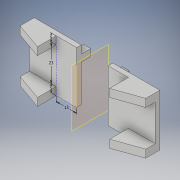
# Autodesk Inventor part: turret_servo_grip
Saved by Autodesk Inventor 2019 (Build 230136000, 136)
## iProperties
Created: 2019-04-21
Part Number: turret_servo_grip
Material: Ogólny
Document SubType Name: Modeling
Designer: terg
Density: 1 g/cm^3
Appearance: Domyślna
Author: terg
Autodesk Inventor part; units mm, degrees
ref_plane "XZ Plane" through (0, 0, 0) normal (0, 1, 0) x (-1, 0, 0)
ref_plane "XY Plane" through (0, 0, 0) normal (0, 0, 1) x (1, 0, 0)
sketch "Szkic1" plane through (0, 0, 0) normal (0, 0, 1) x (1, 0, 0)
  point P0 (0, 0)
sketch "Szkic2" plane through (0, 0, 0) normal (0, 0, 1) x (1, 0, 0)
  line L0 (0, 0) -> (-4.5, 0)
  line L1 (-4.5, 0) -> (-4.5, 4.5)
  line L2 (-4.5, 4.5) -> (0, 4.5)
  line L3 (0, 4.5) -> (0, 0)
  dimension "d0" = 4.5
  dimension "d1" = 4.5
  constraints: 8 end point, 2 parallel, 1 horizontal, 1 perpendicular
  measures "d0" distance of L1.end L2.end
  measures "d1" distance of L0.end L1.end
extrude "Wyciągnięcie proste1" add sketch "Szkic2" along normal blind 6
sketch "Szkic3" plane through (0, 0, 6) normal (0, 0, 1) x (1, 0, 0)
  line L0 (0, 0) -> (0, 4.5) projected
  line L1 (0, 4.5) -> (0, 9.5)
  line L2 (0, 9.5) -> (-30, 9.5)
  line L3 (-30, 9.5) -> (-30, -23.5)
  line L4 (-30, -23.5) -> (0, -23.5)
  line L5 (0, -23.5) -> (0, 9.5)
  point P0 (-4.5, 0)
  dimension "d7" = 5
  dimension "d8" = 30
  dimension "d9" = 33
  constraints: 10 end point, 2 parallel, 1 horizontal, 1 perpendicular, 1 vertical
  measures "d7" distance of L0.end L1.end
  measures "d8" distance of L4.end L3.end
  measures "d9" distance of L3.end L2.end
extrude "Wyciągnięcie proste2" add sketch "Szkic3" along normal blind 3
sketch "Szkic4" plane through (0, 0, 9) normal (0, 0, 1) x (1, 0, 0)
  line L0 (0, -23.5) -> (0, 0) construction
  line L1 (0, -23.5) -> (-13, -23.5) construction
  line L2 (-30, -23.5) -> (0, -23.5) construction
  line L3 (-13, -23.5) -> (-13, -18.5) construction
  line L4 (-13, -18.5) -> (-13, 4.5) construction
  line L5 (-13, 4.5) -> (-13, 9.5) construction
  dimension "d12" = 13
  dimension "d13" = 5
  dimension "d14" = 23
  dimension "d15" = 5
  constraints: 8 end point, 3 vertical, 1 point on line
  measures "d12" distance of L0.start L1.end
  measures "d13" distance of L1.end L3.end
  measures "d14" distance of L3.end L4.end
  measures "d15" distance of L4.end L5.end
sketch "Szkic5" plane through (0, 0, 9) normal (0, 0, 1) x (1, 0, 0)
  line L0 (-30, 9.5) -> (-30, -23.5) projected
  line L1 (-13, -23.5) -> (-30, -23.5)
  line L2 (-30, -23.5) -> (-30, -18.5)
  line L3 (-30, -18.5) -> (-13, -18.5)
  line L4 (-13, -18.5) -> (-13, -23.5)
  line L5 (-13, 4.5) -> (-30, 4.5)
  line L6 (-30, 4.5) -> (-30, 9.5)
  line L7 (-30, 9.5) -> (-13, 9.5)
  line L8 (-13, 9.5) -> (-13, 4.5)
  point P0 (0, 0)
  point P1 (-13, 9.5)
  constraints: 16 end point, 4 parallel, 2 horizontal, 2 perpendicular, 1 point on line
extrude "Wyciągnięcie proste3" add sketch "Szkic5" along normal blind 12
sketch "Szkic6" plane through (-30, -23.5, 6) normal (0, -1, 0) x (1, 0, 0)
  line L0 (17, 15) -> (0, 15) construction
  line L1 (0, 15) -> (0, 9) construction
  line L2 (0, 0) -> (0, 15) construction
  line L3 (17, 15) -> (0, 9)
  arc A0 (17, 15) -> (0, 9) centre (7.5523, 14.6851) ccw
  point P0 (30, -6)
  dimension "d18" = 6
  constraints: 4 end point, 2 point on circle, 1 centre point, 1 point on line
  measures "d18" distance of L0.end L1.end
extrude "Wyciągnięcie proste4" cut sketch "Szkic6" against normal blind 33
ref_plane "Płaszczyzna konstrukcyjna1" through (10, 0, 0) normal (1, 0, 0) x (0, 1, 0)
mirror "Odbij1" about plane through (10, 0, 0) normal (1, 0, 0)
